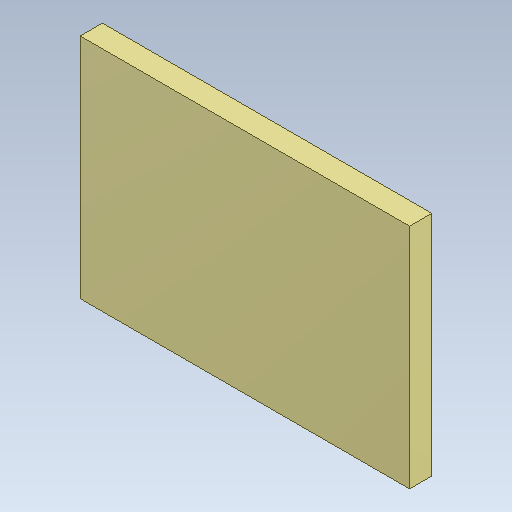
# Autodesk Inventor part: SAMTEC-FTSH-105-01-X-DVJ
Saved by Autodesk Inventor 2021 (Build 250183000, 183)
## iProperties
Created: 2020-11-03
Part Number: SAMTEC-FTSH-105-01-X-DVJ
Material: Generic
Document SubType Name: Modeling
Designer: faiya
Density: 1 g/cm^3
Appearance: SAMTEC-FTSH-105-01-X-DV, SAMTEC-FTSH-105-01-X-DVJ
Author: faiya
Autodesk Inventor part; units mm, degrees
ref_plane "YZ Plane" through (0, 0, 0) normal (1, 0, 0) x (0, 1, 0)
ref_plane "XZ Plane" through (0, 0, 0) normal (0, 1, 0) x (-1, 0, 0)
ref_plane "XY Plane" through (0, 0, 0) normal (0, 0, 1) x (1, 0, 0)
sketch "SAMTEC-FTSH-105-01-X-DV, SAMTEC-FTSH-105-01-X-DVJ_8" plane through (0, 0, 0) normal (0, 0, 1) x (1, 0, 0)
  line L0 (-10.099, 6.128) -> (4.731, 6.128)
  line L1 (4.731, 6.128) -> (4.731, -4.113)
  line L2 (4.731, -4.113) -> (-10.099, -4.113)
  line L3 (-10.099, -4.113) -> (-10.099, 6.128)
  constraints: 8 end point
extrude "Extrusion1" add sketch "SAMTEC-FTSH-105-01-X-DV, SAMTEC-FTSH-105-01-X-DVJ_8" along normal blind 1
body "Solid1"
